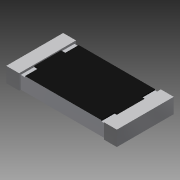
# Autodesk Inventor part: 2020Resistor
Saved by Autodesk Inventor 2014 (Build 180170000, 170)
## iProperties
Created: 2015-11-06
Part Number: 2020Resistor
Material: Generic
Document SubType Name: Modeling
Designer: Owner
Density: 1 g/cm^3
Appearance: Default
Author: Owner
Autodesk Inventor part; units mm, degrees
ref_plane "YZ Plane" through (0, 0, 0) normal (1, 0, 0) x (0, 1, 0)
ref_plane "XZ Plane" through (0, 0, 0) normal (0, 1, 0) x (-1, 0, 0)
ref_plane "XY Plane" through (0, 0, 0) normal (0, 0, 1) x (1, 0, 0)
sketch "Sketch1" plane through (0, 0, 0) normal (0, 1, 0) x (-1, 0, 0)
  line L0 (-2.3198, 1.3198) -> (2.6802, 1.3198)
  line L1 (2.6802, 1.3198) -> (2.6802, -1.1802)
  line L2 (2.6802, -1.1802) -> (-2.3198, -1.1802)
  line L3 (-2.3198, -1.1802) -> (-2.3198, 1.3198)
  point P0 (0, 0)
  dimension "d0" = 5
  dimension "d1" = 2.5
  constraints: 8 end point, 2 parallel, 1 horizontal, 1 perpendicular
  measures "d0" distance of L0.start L0.end
  measures "d1" distance of L0.end L1.end
extrude "Extrusion1" add sketch "Sketch1" along normal blind 0.6
sketch "Sketch2" plane through (0, 0, 0) normal (0, -1, 0) x (1, 0, 0)
  line L0 (-2.6802, -1.1802) -> (2.3198, -1.1802) projected
  line L1 (2.3198, -1.1802) -> (2.3198, 1.3198) projected
  line L2 (-2.7552, 1.3948) -> (-2.1552, 1.3948)
  line L3 (-2.1552, 1.3948) -> (-2.1552, -1.2552)
  line L4 (-2.1552, -1.2552) -> (-2.7552, -1.2552)
  line L5 (-2.7552, -1.2552) -> (-2.7552, 1.3948)
  line L6 (2.3948, -1.2552) -> (1.7948, -1.2552)
  line L7 (1.7948, -1.2552) -> (1.7948, 1.3948)
  line L8 (1.7948, 1.3948) -> (2.3948, 1.3948)
  line L9 (2.3948, 1.3948) -> (2.3948, -1.2552)
  point P0 (0, 0)
  dimension "d4" = 0.6
  dimension "d5" = 0.6
  dimension "d6" = 5.15
  dimension "d7" = 0.075
  dimension "d8" = 2.65
  dimension "d9" = 2.65
  dimension "d11" = 0.075
  dimension "d12" = 0.075
  constraints: 16 end point, 4 parallel, 2 horizontal, 2 perpendicular
  measures "d4" distance of L2.start L2.end
  measures "d5" distance of L7.end L8.end
  measures "d6" distance between parallel lines of L9 L5
  measures "d7" distance between parallel lines of L1 L9
  measures "d8" distance of L4.end L2.start
  measures "d9" distance of L8.end L6.start
  measures "d11" distance between parallel lines of L6 L0
  measures "d12" distance between parallel lines of L0 L4
extrude "Extrusion2" add sketch "Sketch2" against normal blind 0.7
sketch "Sketch3" plane through (0, 0.6, 0) normal (0, 1, 0) x (1, 0, 0)
  line L0 (1.7948, -1.3198) -> (1.7948, 1.1802) projected
  line L1 (1.7948, 1.1802) -> (-2.1552, 1.1802) projected
  line L2 (-2.1552, 1.1802) -> (1.7948, 1.1802)
  line L3 (1.7948, 1.1802) -> (1.7948, -1.3198)
  line L4 (1.7948, -1.3198) -> (-2.1552, -1.3198)
  line L5 (-2.1552, -1.3198) -> (-2.1552, 1.1802)
  line L6 (-2.1552, 1.1802) -> (-1.9552, 1.1802)
  line L7 (-1.9552, 1.1802) -> (-1.9552, 0.5552)
  line L8 (-1.9552, 0.5552) -> (-2.1552, 0.5552)
  line L9 (-2.1552, 0.5552) -> (-2.1552, 1.1802)
  line L10 (-2.1552, -1.3198) -> (-1.9552, -1.3198)
  line L11 (-1.9552, -1.3198) -> (-1.9552, -0.6948)
  line L12 (-1.9552, -0.6948) -> (-2.1552, -0.6948)
  line L13 (-2.1552, -0.6948) -> (-2.1552, -1.3198)
  line L14 (1.7948, 1.1802) -> (1.5948, 1.1802)
  line L15 (1.5948, 1.1802) -> (1.5948, 0.5552)
  line L16 (1.5948, 0.5552) -> (1.7948, 0.5552)
  line L17 (1.7948, 0.5552) -> (1.7948, 1.1802)
  line L18 (1.7948, -1.3198) -> (1.5948, -1.3198)
  line L19 (1.5948, -1.3198) -> (1.5948, -0.6948)
  line L20 (1.5948, -0.6948) -> (1.7948, -0.6948)
  line L21 (1.7948, -0.6948) -> (1.7948, -1.3198)
  point P0 (0, 0)
  dimension "d15" = 0.2
  dimension "d16" = 0.2
  dimension "d17" = 0.2
  dimension "d18" = 0.2
  dimension "d19" = 0.625
  dimension "d20" = 0.625
  dimension "d21" = 0.625
  dimension "d22" = 0.625
  constraints: 40 end point, 10 parallel, 5 horizontal, 5 perpendicular
  measures "d15" distance of L7.end L8.end
  measures "d16" distance of L15.end L16.end
  measures "d17" distance of L19.end L20.end
  measures "d18" distance of L11.end L12.end
  measures "d19" distance of L10.end L11.end
  measures "d20" distance of L6.end L7.end
  measures "d21" distance of L14.end L15.end
  measures "d22" distance of L18.end L19.end
extrude "Extrusion3" add sketch "Sketch3" along normal blind 0.05 contours L20 L19 L4 L11 L12 L5 L8 L7 L1 L15 L16 L0
body "Solid1"
